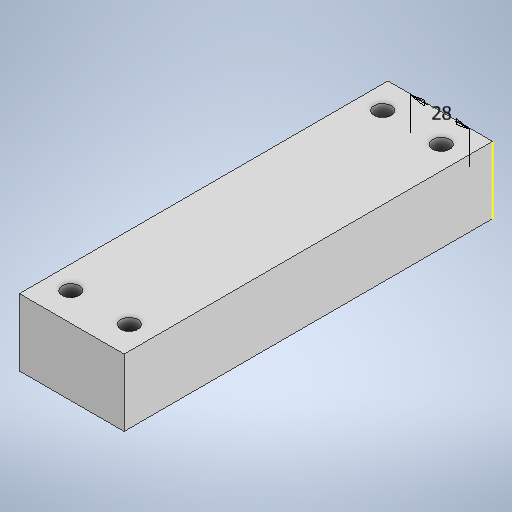
# Autodesk Inventor part: 13042026-05
Saved by Autodesk Inventor 2025.2 (Build 292293000, 293)
## iProperties
Created: 2026-05-05
Part Number: 13042026-05
Material: Generic
Document SubType Name: Modeling
Designer: Oski
Density: 1 g/cm^3
Appearance: Default
Author: Oski
Autodesk Inventor part; units mm, degrees
ref_plane "YZ Plane" through (0, 0, 0) normal (1, 0, 0) x (0, 1, 0)
ref_plane "XZ Plane" through (0, 0, 0) normal (0, 1, 0) x (-1, 0, 0)
ref_plane "XY Plane" through (0, 0, 0) normal (0, 0, 1) x (1, 0, 0)
sketch "Sketch2" plane through (0, 0, 0) normal (0, 0, 1) x (1, 0, 0)
  line L0 (-25, 16) -> (25, 16)
  line L1 (25, 16) -> (25, -16)
  line L2 (25, -16) -> (-25, -16)
  line L3 (-25, -16) -> (-25, 16)
  line L4 (-25, 16) -> (25, -16) construction
  line L5 (25, 16) -> (-25, -16) construction
  point P0 (0, 0)
  dimension "d4" = 32
  dimension "d5" = 50
  constraints: 12 end point, 2 midpoint, 2 parallel, 1 horizontal, 1 perpendicular
  measures "d4" distance of L0.end L1.end
  measures "d5" distance of L1.end L2.end
extrude "Extrusion1" add sketch "Sketch2" along normal mid plane 176
sketch "Sketch5" plane through (0, 0, -88) normal (0, 0, -1) x (-1, 0, 0)
  line L0 (-14, 0) -> (-25, 0) construction
  line L1 (-25, -16) -> (-25, 16) projected
  line L2 (14, 0) -> (25, 0) construction
  line L3 (25, 16) -> (25, -16) projected
  line L4 (-25, 0) -> (25, 0) construction
  point P0 (0, 0)
  dimension "d14" = 28
  constraints: 6 end point, 2 midpoint, 2 point on line, 1 collinear, 1 horizontal
  measures "d14" distance of L0.start L2.start
sketch "Sketch6" plane through (-25, -16, -88) normal (0, -1, 0) x (1, 0, 0)
  point P0 (25, 88)
sketch "Sketch9" plane through (-25, -16, 88) normal (0, -1, 0) x (1, 0, 0)
  line L0 (0, 0) -> (50, 0) projected
  line L1 (39, 0) -> (39, -176) construction
  line L2 (0, -176) -> (50, -176) projected
  line L3 (50, -176) -> (0, -176) construction
  line L4 (39, -13.5) -> (50, -13.5) construction
  line L5 (50, -176) -> (50, 0) construction
  line L6 (11, -13.5) -> (0, -13.5) construction
  line L7 (0, 0) -> (0, -176) construction
  line L8 (11, -13.5) -> (11, 0)
  line L9 (11, -162.5) -> (0, -162.5) construction
  line L10 (11, -162.5) -> (11, -176) construction
  point P0 (25, -88)
  point P1 (39, -162.5)
  dimension "d36" = 28
  dimension "d37" = 28
  dimension "d38" = 149
  constraints: 12 end point, 10 point on line, 4 perpendicular, 3 equal length, 1 collinear, 1 vertical
  measures "d36" distance of L6.start L4.start
  measures "d37" distance of point (39, -162.5) L9.start
  measures "d38" distance of point (39, -162.5) L4.start
hole "Hole3" at (14, -16, 74.5) at (-14, -16, 74.5) at (14, -16, -74.5) at (-14, -16, -74.5) direction (0, 1, 0) diameter 8.2 end through all
body "Solid1"
